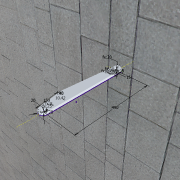
# Autodesk Inventor part: Profile_Straight
Saved by Autodesk Inventor 2016 (Build 200138000, 138)
## iProperties
Created: 2015-05-19
Part Number: Profile_Straight
Material: Aluminum 6061
Document SubType Name: Modeling
Designer: Yann
Density: 2.7 g/cm^3
Appearance: Aluminum - Flat
Mass: 986.272 g
Surface Area: 982.77 cm^2
Volume: 365.286 cm^3
Author: Yann
Autodesk Inventor part; units mm, degrees
ref_plane "YZ Plane" through (0, 0, 0) normal (1, 0, 0) x (0, 1, 0)
ref_plane "XZ Plane" through (0, 0, 0) normal (0, 1, 0) x (-1, 0, 0)
ref_plane "XY Plane" through (0, 0, 0) normal (0, 0, 1) x (1, 0, 0)
sketch "Sketch2" plane through (0, 0, 0) normal (0, 1, 0) x (-1, 0, 0)
  circle A0 centre (0, 490) radius 10
  circle A1 centre (0, 0) radius 10
  line L0 (24.5876, 494.5222) -> (49.3695, 359.7814)
  line L1 (50.7256, 334.0357) -> (21.9944, -40.0968)
  line L2 (18.9282, -41.6321) -> (-24.072, -14.3293)
  line L3 (-25, -12.6409) -> (-25, 490)
  arc A2 (24.5876, 494.5222) -> (-25, 490) centre (0, 490) ccw
  line L4 (0, -154.4311) -> (0, 629.0893) construction
  arc A3 (18.9282, -41.6321) -> (21.9944, -40.0968) centre (20.0003, -39.9437) ccw
  arc A4 (-25, -12.6409) -> (-24.072, -14.3293) centre (-23, -12.6409) ccw
  arc A5 (50.7256, 334.0357) -> (49.3695, 359.7814) centre (-48.9808, 341.6925) ccw
  line L5 (-17, 19.4683) -> (-17, 467.2676)
  line L6 (43.2667, 341.388) -> (18.4452, 18.1672)
  line L7 (15.4511, 16.5882) -> (5, 22.6222)
  line L8 (4, 24.3542) -> (4, 456.3028)
  line L9 (4.5133, 457.6406) -> (17.3407, 471.896)
  line L10 (-13.6891, 468.7781) -> (-4.6891, 460.9668)
  line L11 (-4, 459.4563) -> (-4, 27.5077)
  line L12 (-4.6676, 26.0162) -> (-13.6676, 17.9767)
  line L13 (-69.1212, 0) -> (71.8613, 0) construction
  line L14 (20.7944, 470.92) -> (42.7242, 351.6863)
  arc A6 (43.2667, 341.388) -> (42.7242, 351.6863) centre (3.3841, 344.4507) ccw
  arc A7 (-17, 19.4683) -> (-13.6676, 17.9767) centre (-15, 19.4683) ccw
  arc A8 (-4.6676, 26.0162) -> (-4, 27.5077) centre (-6, 27.5077) ccw
  arc A9 (4, 24.3542) -> (5, 22.6222) centre (6, 24.3542) ccw
  arc A10 (15.4511, 16.5882) -> (18.4452, 18.1672) centre (16.4511, 18.3203) ccw
  arc A11 (4.5133, 457.6406) -> (4, 456.3028) centre (6, 456.3028) ccw
  arc A12 (20.7944, 470.92) -> (17.3407, 471.896) centre (18.8274, 470.5582) ccw
  arc A13 (-13.6891, 468.7781) -> (-17, 467.2676) centre (-15, 467.2676) ccw
  arc A14 (-4, 459.4563) -> (-4.6891, 460.9668) centre (-6, 459.4563) ccw
  circle A15 centre (24.5876, 339.2417) radius 4
  circle A16 centre (-9.1676, 339.2417) radius 4
  point P0 (51.7209, 346.9967)
  point P1 (-17, 15)
  point P2 (18.202, 15)
  dimension "d0" = 20
  dimension "d1" = 20
  dimension "d2" = 490
  dimension "d3" = 15
  dimension "d4" = 10.421
  dimension "d6" = 25
  dimension "d7" = 25
  dimension "d8" = 25
  dimension "d9" = 150
  dimension "d10" = 2
  dimension "d11" = 100
  dimension "d14" = 15
  dimension "d15" = 15
  dimension "d16" = 8
  dimension "d18" = 8
  dimension "d19" = 8
  dimension "d20" = 60
  dimension "d21" = 40
  dimension "d22" = 8
  dimension "d23" = 25
  dimension "d24" = 25
  dimension "d25" = 2
  dimension "d28" = 8
  constraints: 27 point on circle, 26 end point, 26 tangent, 17 centre point, 9 equal radius, 8 point on line, 3 parallel, 2 coincident, 2 equal length, 1 vertical, 1 other
  measures "d0" diameter of A0
  measures "d1" diameter of A1
  measures "d2" distance of point (0, 0) A0.centre
  measures "d3" radial gap between concentric circles of A2 A0
  measures "d4" angle of L0 L4
  measures "d6" distance from line of L3 A1.centre
  measures "d7" distance from line of A1.centre L2
  measures "d8" distance from line of A1.centre L1
  measures "d9" distance of L0.start point (51.721, 346.997)
  measures "d10" radius of A3
  measures "d11" radius of A5
  measures "d14" distance from line of L13 point (-17, 15)
  measures "d15" distance from line of L13 point (18.202, 15)
  measures "d16" distance between parallel lines of L3 L5
  measures "d18" distance between parallel lines of L1 L6
  measures "d19" distance between parallel lines of L8 L11
  measures "d20" angle of L4 L7
  measures "d21" radius of A6
  measures "d22" distance between parallel lines of L0 L14
  measures "d23" distance from line of A0.centre L9
  measures "d24" distance from line of L10 A0.centre
  measures "d25" radius of A7
  measures "d28" diameter of A16
extrude "Extrusion1" add sketch "Sketch2" along normal blind 15 contours L0 A5 L1 A3 L2 A4 L3 A2 | L5 A13 L10 A14 L11 A8 L12 A7 | L6 A10 L7 A9 L8 A11 L9 A12 L14 A6
extrude "Extrusion2" cut sketch "Sketch2" along normal blind 7 contours L5 A13 L10 A14 L11 A8 L12 A7 | L6 A10 L7 A9 L8 A11 L9 A12 L14 A6 | A15 | A16
equation "\"d1\" = d0"
equation "\"d6\" = 0.5 * d1 + d3"
equation "\"d7\" = d6"
equation "\"d8\" = d6"
equation "\"d15\" = d14"
equation "\"d18\" = d16"
equation "\"d19\" = d16"
equation "\"d22\" = d16"
equation "\"d23\" = 0.5 * d0 + d3"
equation "\"d24\" = d23"
body "Solid1"
